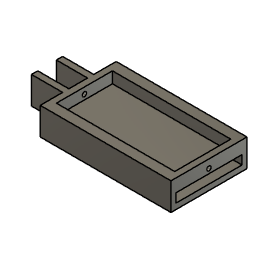
ManipulateurCW v3 (Autodesk Fusion 360 design; units mm, degrees)
Autodesk Fusion 360 part; units mm, degrees
box "BoitePrimitive1" add length 20 width 55 height 100 placed x (0, 1, 0) y (0, 0, 1) z (1, 0, 0) at (0, 0, -30) makes body 1
box "BoitePrimitive2" cut length 5.2 width 50 height 100 placed x (0, 1, 0) y (0, 0, 1) z (1, 0, 0) at (0, 2.499, -27.5321) bodies 1
box "BoitePrimitive3" add length 10 width 45 height 90 placed x (0, -1, 0) y (0, 0, -1) z (1, 0, 0) at (0, 20, 20) separate body makes body 2
move_face "DéplacerFace1" by (0, -5, 0) 1 faces at (0, 16.6667, -10) on bodies 2
move_body "Déplacer1" bodies 1 to x (1, 0, 0) y (0, 1, 0) z (0, 0, 1) at (-5, 0, 0)
combine "Combiner1" operation cut target body 1 tool bodies 2
cylinder "CylindrePrimitive1" cut diameter 3.5 height -10 placed x (0, 0, -1) y (0, 1, 0) z (1, 0, 0) at (95, 13.3864, -2.5) bodies 1
move_face "DéplacerFace2" by (-5, 0, 0) 1 faces at (-5, 15.8997, 5.8226) on bodies 1
move_face "DéplacerFace3" by (-5, 0, 0) 1 faces at (0, 16.6667, -10) on bodies 1
box "BoitePrimitive5" add length 5.2 width 50 height -4 placed x (0, 1, 0) y (0, 0, -1) z (-1, 0, 0) at (-10, 2.499, 22.4679) bodies 1
box "BoitePrimitive7" add length 20 width 3 height 15 placed x (0, 1, 0) y (0, 0, -1) z (-1, 0, 0) at (-10, 0, -5) bodies 1
box "BoitePrimitive8" add length 20 width 3 height 15 placed x (0, 1, 0) y (0, 0, -1) z (-1, 0, 0) at (-10, 0, 8) bodies 1
move_face "DéplacerFace6" by (0, 0, -2) 1 faces at (-15, 13.3333, -8) on bodies 1
move_face "DéplacerFace7" by (0, 0, -1) 1 faces at (-15, 13.3333, -5) on bodies 1
move_face "DéplacerFace8" by (0, 0, 3) 1 faces at (-15, 13.3333, 8) on bodies 1
move_face "DéplacerFace9" by (0, 0, 2) 1 faces at (-15, 13.3333, 5) on bodies 1
move_face "DéplacerFace10" by (0, 0, -4) 1 faces at (-15, 13.3333, 7) on bodies 1
move_face "DéplacerFace11" by (0, 0, -6) 1 faces at (-15, 13.3333, 11) on bodies 1
move_face "DéplacerFace12" by (0, 0, -2) 1 faces at (-15, 13.3333, 3) on bodies 1
cylinder "CylindrePrimitive5" cut diameter 3.5 height -10 placed x (0, 0, 1) y (0, 1, 0) z (-1, 0, 0) at (-10, 14.9777, -2.5521) bodies 1
move_face "DéplacerFace13" by (0, 0, 0.5) 1 faces at (61.3333, 4.2324, 22.4679) on bodies 1
move_face "DéplacerFace14" by (0, 0, -0.5) 1 faces at (61.3333, 4.2324, -27.5321) on bodies 1
move_face "DéplacerFace15" by (0, -2, 0) 1 faces at (60, 0, -1.3333) on bodies 1
move_face "DéplacerFace16" by (0, 2, 0) 1 faces at (27.6667, 7.699, -11.0321) on bodies 1
move_face "DéplacerFace17" by (0, 0, 2) 1 faces at (25, 5.3333, 25) on bodies 1
move_face "DéplacerFace18" by (0, 0, -2) 1 faces at (25, 5.3333, -30) on bodies 1
move_face "DéplacerFace19" by (0, 0, 1) 1 faces at (27.6667, 7.299, 22.9679) on bodies 1
move_face "DéplacerFace20" by (0, 0, -1) 1 faces at (61.3333, 4.899, -28.0321) on bodies 1
move_face "DéplacerFace21" by (0, 0, 1) 1 faces at (25, 5.3333, 27) on bodies 1
move_face "DéplacerFace22" by (0, 0, -1) 1 faces at (25, 5.3333, -32) on bodies 1
move_face "DéplacerFace23" by (0, 0, -5) 1 faces at (-15, 12.6667, -10) on bodies 1
move_face "DéplacerFace24" by (0, 0, -4) 1 faces at (-15, 12.6667, -6) on bodies 1
move_face "DéplacerFace25" by (0, 0, 5) 1 faces at (-15, 12.6667, 5) on bodies 1
move_face "DéplacerFace26" by (0, 0, 4) 1 faces at (-15, 12.6667, 1) on bodies 1
move_face "DéplacerFace27" by (0, 1, 0) 1 faces at (26.6667, 10, -10) on bodies 1
move_face "DéplacerFace28" by (-15, 0, 0) 1 faces at (-25, 5.3333, 6.6667) on bodies 1
move_face "DéplacerFace29" by (5, 0, 0) 1 faces at (-40, 5.3333, 6.6667) on bodies 1
move_face "DéplacerFace30" by (-10, 0, 0) 1 faces at (-25, 12.6667, -11.6667) on bodies 1
